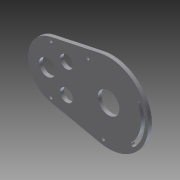
# Autodesk Inventor part: front plate
Saved by Autodesk Inventor 2012 (Build 160160000, 160)
## iProperties
Created: 2012-01-30
Part Number: front plate
Material: Default
Document SubType Name: Modeling
Designer: Antonella Wilby
Density: 1 g/cm^3
Author: Antonella Wilby
Autodesk Inventor part; units mm, degrees
ref_plane "YZ Plane" through (0, 0, 0) normal (1, 0, 0) x (0, 1, 0)
ref_plane "XZ Plane" through (0, 0, 0) normal (0, 1, 0) x (-1, 0, 0)
ref_plane "XY Plane" through (0, 0, 0) normal (0, 0, 1) x (1, 0, 0)
sketch "Sketch1" plane through (0, 0, 0) normal (0, 0, 1) x (1, 0, 0)
  line L0 (-184.0318, 0) -> (112.1636, 0) projected
  line L1 (0, -97.79) -> (0, 97.79) projected
  circle A0 centre (0, 0) radius 50.8 construction
  arc A1 (-14.6356, -68.2995) -> (-14.6356, 68.2995) centre (0, 0) ccw
  arc A2 (44.9013, -44.9013) -> (57.5505, 26.8363) centre (0, 0) ccw
  arc A3 (40.1305, -40.1305) -> (51.4358, 23.9849) centre (0, 0) ccw
  line L2 (0, 0) -> (57.5505, 26.8363) construction
  line L3 (0, 0) -> (44.9013, -44.9013) construction
  arc A4 (57.5505, 26.8363) -> (51.4358, 23.9849) centre (54.4932, 25.4106) ccw
  arc A5 (40.1305, -40.1305) -> (44.9013, -44.9013) centre (42.5159, -42.5159) ccw
  arc A6 (-101.5622, 49.6724) -> (-101.5622, -49.6724) centre (-90.9182, 0) ccw
  line L4 (-101.5622, 49.6724) -> (-14.6356, 68.2995)
  line L5 (-101.5622, -49.6724) -> (-14.6356, -68.2995)
  circle A7 centre (-74.0404, 25.4) radius 11.1125
  circle A8 centre (-74.0404, -25.4) radius 11.1125
  circle A9 centre (0, 0) radius 19.05
  circle A10 centre (-107.95, 0) radius 14.2875
  line L6 (-107.95, -14.2875) -> (-107.95, 14.2875) construction
  dimension "d0" = 101.6
  dimension "d1" = 19.05
  dimension "d2" = 6.7469
  dimension "d3" = 6.35
  dimension "d4" = 45
  dimension "d5" = 25
  dimension "d10" = 22.225
  dimension "d11" = 38.1
  dimension "d24" = 50.8
  dimension "d33" = 88.9
  dimension "d34" = 107.95
  dimension "d35" = 28.575
  constraints: 14 point on circle, 11 centre point, 10 end point, 6 tangent, 3 coincident, 3 point on line, 1 horizontal alignment, 1 midpoint, 1 parallel, 1 symmetric about line, 1 other
  measures "d0" diameter of A0
  measures "d1" radial gap between concentric circles of A1 A0
  measures "d2" radial gap between concentric circles of A2 A3
  measures "d3" radial gap between concentric circles of A1 A2
  measures "d4" angle of L0 L3
  measures "d5" angle of L2 L0
  measures "d10" diameter of A7
  measures "d11" diameter of A9
  measures "d24" radius of A6
  measures "d33" distance of L4.start L4.end
  measures "d34" distance between parallel lines of L1 L6
  measures "d35" diameter of A10
extrude "Extrusion1" add sketch "Sketch1" along normal mid plane 6.35 contours A6 L4 A1 L1 A9 L0 A10 | L0 A10 A9 L1 A1 L5 A6 | A1 L0 A2 A4 A3 A9 L1 | L1 A9 L0 A3 A5 A2 A1
sketch "Sketch2" plane through (0, 0, -3.175) normal (0, 0, -1) x (-1, 0, 0)
  line L0 (184.0318, 0) -> (-112.1636, 0) projected
  line L1 (0, -97.79) -> (0, 97.79) projected
  point P0 (36.5125, 49.2125)
  point P1 (9.525, -60.325)
  dimension "d15" = 49.2125
  dimension "d16" = 36.5125
  dimension "d39" = 9.525
  dimension "d40" = 60.325
  measures "d15" distance from line of L0 point (36.513, 49.212)
  measures "d16" distance from line of L1 point (36.513, 49.212)
  measures "d39" distance from line of L1 point (9.525, -60.325)
  measures "d40" distance from line of L0 point (9.525, -60.325)
hole "Hole1" at (-36.5125, 49.2125, -3.175) at (-9.525, -60.325, -3.175) direction (0, 0, 1) diameter 5.1054 end through all counterbore diameter 9.779 counterbore depth 1.5875 clearance for "Flat Head Machine Screw (82)" size "#10" standard "Ansi Unified Screw Threads"
sketch "Sketch3" plane through (0, 0, -3.175) normal (0, 0, -1) x (-1, 0, 0)
  line L0 (101.5622, -49.6724) -> (101.5622, 49.6724) construction
  line L1 (184.0318, 0) -> (-112.1636, 0) projected
  line L2 (0, -97.79) -> (0, 97.79) projected
  point P0 (101.5622, 42.8625)
  point P1 (101.5622, -42.8625)
  dimension "d25" = 42.8625
  constraints: 2 end point, 1 point on line, 1 symmetric about line, 1 vertical
  measures "d25" distance from line of point (101.562, 42.862) L1
hole "Hole2" at (-101.5622, 42.8625, -3.175) at (-101.5622, -42.8625, -3.175) direction (0, 0, 1) diameter 5.1054 end through all counterbore diameter 9.779 counterbore depth 1.5875 clearance for "Flat Head Machine Screw (82)" size "#10" standard "Ansi Unified Screw Threads"
body "Solid1"
